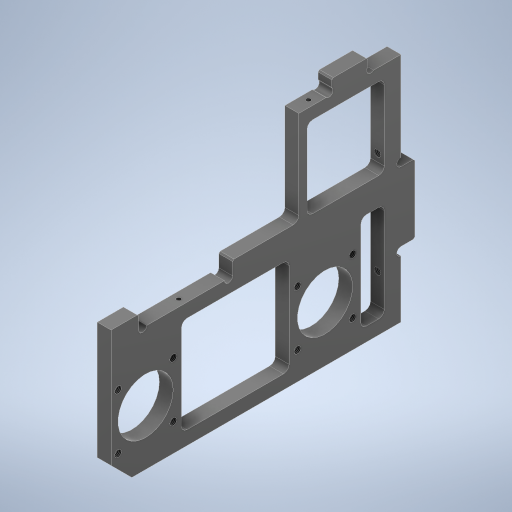
# Autodesk Inventor part: TorsoElectronicBoxSideFrame_
Saved by Autodesk Inventor 2024.2 (Build 282272000, 272)
## iProperties
Created: 2024-01-27
Part Number: TorsoElectronicBoxSideFrame_
Material: Acetal Resin, Black
Document SubType Name: Modeling
Designer: Masato Kubotera
Density: 1.425 g/cm^3
Appearance: Smooth - Black
Vendor: meviy
Mass: 35.6597 g
Surface Area: 137.332 cm^2
Volume: 25.0244 cm^3
Author: Masato Kubotera
Autodesk Inventor part; units mm, degrees
ref_plane "YZ Plane" through (0, 0, 0) normal (1, 0, 0) x (0, 1, 0)
ref_plane "XZ Plane" through (0, 0, 0) normal (0, 1, 0) x (-1, 0, 0)
ref_plane "XY Plane" through (0, 0, 0) normal (0, 0, 1) x (1, 0, 0)
derived "TorsoSideFrame.ipt"
sketch "Sketch1" plane through (0, 0, 0) normal (0, 1, 0) x (-1, 0, 0)
  circle A0 centre (0, 0) radius 18.75
  line L0 (0, 0) -> (0, -161.5)
  circle A1 centre (0, 0) radius 29 construction
  line L1 (0, 0) -> (0, 36)
  line L2 (0, 36) -> (-48.2759, 36)
  line L3 (-65, -12.5) -> (-65, -106.5)
  line L4 (-50, -161.5) -> (-35, -161.5)
  line L5 (-35, -161.5) -> (-35, -166.5)
  line L6 (-35, -166.5) -> (-10, -166.5)
  line L7 (-10, -166.5) -> (-10, -161.5)
  line L8 (-10, -161.5) -> (0, -161.5)
  line L9 (-60, -40.225) -> (-65, -40.225)
  line L10 (-44, -161.5) -> (-44, -155.5) construction
  line L11 (-22.5, -166.5) -> (-22.5, -161.5) construction
  arc A2 (-7, -161.5) -> (-10, -161.5) centre (-8.5, -161.5) ccw
  arc A3 (-35, -161.5) -> (-38, -161.5) centre (-36.5, -161.5) ccw
  line L12 (-65, -12.5) -> (-60, -12.5) construction
  line L13 (-60, -12.5) -> (-60, -101.5) construction
  line L14 (-62.5, -12.5) -> (-62.5, -101.5) construction
  line L15 (-70, -66) -> (0, -66) construction
  line L16 (-65, -40.25) -> (-60, -40.25) construction
  arc A4 (-60, -43.225) -> (-60, -40.225) centre (-60, -41.725) ccw
  line L17 (-60, -106.5) -> (0, -106.5) construction
  line L18 (-60, -101.5) -> (0, -101.5) construction
  line L19 (-60, -104) -> (-18.75, -104) construction
  line L20 (-9.95, -106.55) -> (-27.55, -106.55)
  line L21 (-27.55, -106.55) -> (-27.55, -101.45)
  line L22 (-27.55, -101.45) -> (-9.95, -101.45)
  line L23 (-9.95, -101.45) -> (-9.95, -106.55)
  line L24 (-9.95, -106.55) -> (-27.55, -101.45) construction
  line L25 (-27.55, -106.55) -> (-9.95, -101.45) construction
  line L26 (-27.5, -101.5) -> (-27.5, -106.5) construction
  arc A5 (-24.55, -101.45) -> (-27.55, -101.45) centre (-26.05, -101.45) ccw
  arc A6 (-27.55, -106.55) -> (-24.55, -106.55) centre (-26.05, -106.55) ccw
  line L27 (-22.5, -71.5) -> (-42.5, -71.5) construction
  line L28 (-42.5, -71.5) -> (-42.5, -91.5) construction
  line L29 (-42.5, -91.5) -> (-22.5, -91.5) construction
  line L30 (-22.5, -91.5) -> (-22.5, -71.5) construction
  line L31 (-22.5, -71.5) -> (-42.5, -91.5) construction
  line L32 (-42.5, -71.5) -> (-22.5, -91.5) construction
  line L33 (-45, -69) -> (-20, -69)
  line L34 (-20, -69) -> (-20, -94)
  line L35 (-20, -94) -> (-45, -94)
  line L36 (-45, -94) -> (-45, -69)
  line L37 (-45, -69) -> (-20, -94) construction
  line L38 (-20, -69) -> (-45, -94) construction
  line L39 (-50, 31) -> (0, 31) construction
  line L40 (-38.05, 31.05) -> (-13.95, 31.05)
  line L41 (-13.95, 31.05) -> (-13.95, 25.95)
  line L42 (-13.95, 25.95) -> (-38.05, 25.95)
  line L43 (-38.05, 25.95) -> (-38.05, 31.05)
  line L44 (-38.05, 31.05) -> (-13.95, 25.95) construction
  line L45 (-13.95, 31.05) -> (-38.05, 25.95) construction
  line L46 (-38.05, 28.5) -> (-13.95, 28.5) construction
  line L47 (-38, 31) -> (-38, 26) construction
  line L48 (-26, 31.05) -> (-26, 25.95) construction
  line L49 (-14, 31) -> (-14, 26) construction
  arc A7 (-35.05, 31.05) -> (-38.05, 31.05) centre (-36.55, 31.05) ccw
  arc A8 (-38.05, 25.95) -> (-35.05, 25.95) centre (-36.55, 25.95) ccw
  arc A9 (-13.95, 31.05) -> (-16.95, 31.05) centre (-15.45, 31.05) ccw
  arc A10 (-16.95, 25.95) -> (-13.95, 25.95) centre (-15.45, 25.95) ccw
  line L50 (-46.0671, -156.5) -> (-3.5, -156.5)
  arc A11 (-47.9578, -155.152) -> (-46.0671, -156.5) centre (-46.0671, -154.5) ccw
  arc A12 (-3.5, -156.5) -> (-1.5, -154.5) centre (-3.5, -154.5) ccw
  line L51 (-56, -100.25) -> (-31.1254, -100.25)
  circle A13 centre (-41.25, -65.25) radius 2 construction
  line L52 (-1.5, -63.25) -> (-56, -63.25)
  line L53 (0, 0) -> (-29, 0) construction
  line L54 (-60, -107.75) -> (-31.1254, -107.75)
  arc A14 (-29.4336, -108.6833) -> (-23.3669, -109.5167) centre (-26.05, -106.55) ccw
  line L55 (-1.5, -154.5) -> (-1.5, -109.75)
  arc A15 (-1.5, -109.75) -> (-3.5, -107.75) centre (-3.5, -109.75) ccw
  arc A16 (-29.4336, -108.6833) -> (-31.1254, -107.75) centre (-31.1254, -109.75) ccw
  circle A17 centre (-33.5, -104) radius 1.75 construction
  arc A18 (-22.0254, -109) -> (-23.3669, -109.5167) centre (-22.0254, -111) ccw
  line L56 (-18.75, -101.45) -> (-18.75, -106.55) construction
  arc A19 (-31.1254, -100.25) -> (-29.4336, -99.3167) centre (-31.1254, -98.25) ccw
  arc A20 (-23.3669, -98.4833) -> (-29.4336, -99.3167) centre (-26.05, -101.45) ccw
  arc A21 (-23.3669, -98.4833) -> (-22.0254, -99) centre (-22.0254, -97) ccw
  line L57 (-10, -101.5) -> (-10, -106.5) construction
  arc A22 (-12.95, -106.55) -> (-9.95, -106.55) centre (-11.45, -106.55) ccw
  arc A23 (-6.3746, -107.75) -> (-8.0664, -108.6833) centre (-6.3746, -109.75) ccw
  arc A24 (-14.1331, -109.5167) -> (-15.4746, -109) centre (-15.4746, -111) ccw
  arc A25 (-14.1331, -109.5167) -> (-8.0664, -108.6833) centre (-11.45, -106.55) ccw
  arc A26 (-9.95, -101.45) -> (-12.95, -101.45) centre (-11.45, -101.45) ccw
  arc A27 (-15.4746, -99) -> (-14.1331, -98.4833) centre (-15.4746, -97) ccw
  arc A28 (-8.0664, -99.3167) -> (-14.1331, -98.4833) centre (-11.45, -101.45) ccw
  arc A29 (-8.0664, -99.3167) -> (-6.3746, -100.25) centre (-6.3746, -98.25) ccw
  line L58 (-22.0254, -99) -> (-15.4746, -99)
  line L59 (-22.0254, -109) -> (-15.4746, -109)
  line L60 (-6.3746, -107.75) -> (-3.5, -107.75)
  line L61 (-6.3746, -100.25) -> (-3.5, -100.25)
  arc A30 (-3.5, -100.25) -> (-1.5, -98.25) centre (-3.5, -98.25) ccw
  line L62 (-41.25, -65.25) -> (-36.25, -65.25) construction
  line L63 (-60, -43.225) -> (-60, -87.275)
  line L64 (-60, -65.25) -> (-65, -65.25) construction
  line L65 (-65, -90.25) -> (-60, -90.25) construction
  arc A31 (-60, -90.275) -> (-60, -87.275) centre (-60, -88.775) ccw
  line L66 (-60, -90.275) -> (-65, -90.275)
  line L67 (-60, -101.5) -> (-65, -101.5) construction
  line L68 (-1.5, -22.4499) -> (-1.5, -63.25)
  line L69 (-56, -67.25) -> (-1.5, -67.25)
  line L70 (-1.5, -67.25) -> (-1.5, -98.25)
  line L71 (-56, -63.25) -> (-56, -45.4999)
  circle A32 centre (-32.5, -81.5) radius 10
  line L72 (-56, -67.25) -> (-56, -100.25)
  circle A33 centre (-32.5, -81.5) radius 11
  arc A34 (-14.0872, 17.5443) -> (-22.2374, 3.4277) centre (0, 0) ccw
  arc A35 (-22.2374, -3.4277) -> (-14.0872, -17.5443) centre (0, 0) ccw
  arc A36 (-8.1502, -20.972) -> (-1.5, -22.4499) centre (0, 0) ccw
  arc A37 (-22.2374, 3.4277) -> (-22.2374, -3.4277) centre (-24.75, 0) ccw
  line L73 (-48.2759, 36) -> (-65, -12.5)
  arc A38 (-42.9869, 36) -> (-50, 31) centre (-42.9869, 28.5817) ccw
  line L74 (-75.1102, 42.6949) -> (-93.0397, -9.3006) construction
  ellipse E0 centre (-84.0749, 16.6972) end of major axis (-76.7401, 37.9681) minor radius 15 construction
  ellipse E1 centre (-84.0749, 16.6972) end of major axis (-93.0397, -9.3006) minor radius 20 construction
  line L75 (-75.1102, 42.6949) -> (-76.7401, 37.9681) construction
  line L76 (-105, 43.5) -> (-105, 11.4504) construction
  line L77 (-84.0749, 16.6972) -> (-58.029, 7.7158) construction
  line L78 (-63.4041, 25.9649) -> (-37.3775, 16.9903) construction
  line L79 (-37.3775, 16.9903) -> (-47.4832, -12.3163) construction
  line L80 (-47.4832, -12.3163) -> (-73.5098, -3.3416) construction
  line L81 (-79.9787, 43.5) -> (-105, 43.5) construction
  line L82 (-45.1768, 19.6797) -> (-55.2826, -9.6269) construction
  circle A39 centre (-47.8663, 11.8804) radius 6.25 construction
  circle A40 centre (-52.5931, -1.8275) radius 6.25 construction
  line L83 (-1, 13.5) -> (-28, 13.5) construction
  line L84 (-28, 13.5) -> (-28, -13.5) construction
  line L85 (-28, -13.5) -> (-1, -13.5) construction
  line L86 (-1, -13.5) -> (-1, 13.5) construction
  line L87 (-1, 13.5) -> (-28, -13.5) construction
  line L88 (-28, 13.5) -> (-1, -13.5) construction
  line L89 (0, -65.25) -> (-65, -65.25) construction
  line L90 (-50, -161.5) -> (-65, -118)
  line L91 (-16.326, 23) -> (-48.5275, 23)
  arc A41 (-16.326, 23) -> (-14.0872, 17.5443) centre (-12.375, 21.4341) ccw
  line L92 (-65, -106.5) -> (-65, -118)
  arc A42 (-56, -45.4999) -> (-60, -36.225) centre (-60, -41.725) ccw
  arc A43 (-46.8371, 5.7157) -> (-50.3902, 17.5981) centre (-47.8663, 11.8804) ccw
  arc A44 (-46.8371, 5.7157) -> (-47.983, 2.3925) centre (-46.5078, 3.743) ccw
  arc A45 (-58.1048, -4.7743) -> (-47.983, 2.3925) centre (-52.5931, -1.8275) ccw
  line L93 (-48.5275, 23) -> (-50.3902, 17.5981)
  line L94 (-38, 26) -> (-14, 26) construction
  line L95 (-58.1048, -4.7743) -> (-60, -10.2703)
  line L96 (-60, -36.225) -> (-60, -10.2703)
  line L97 (-39.0921, -23.3529) -> (-39.0921, -46.6256) construction
  line L98 (-54.0921, -23.3529) -> (-54.0921, -46.6256) construction
  line L99 (-39.0921, -23.3529) -> (-54.0921, -23.3529) construction
  line L100 (-39.0921, -46.6256) -> (-54.0921, -46.6256) construction
  line L101 (-16.326, -23) -> (-48.5275, -23)
  arc A46 (-14.0872, -17.5443) -> (-16.326, -23) centre (-12.375, -21.4341) ccw
  line L102 (-47.9578, -155.152) -> (-50.3902, -148.0981)
  arc A47 (-50.3902, -148.0981) -> (-46.8371, -136.2157) centre (-47.8663, -142.3804) ccw
  arc A48 (-47.983, -132.8925) -> (-46.8371, -136.2157) centre (-46.5078, -134.243) ccw
  arc A49 (-47.983, -132.8925) -> (-58.1048, -125.7257) centre (-52.5931, -128.6725) ccw
  line L103 (-58.1048, -125.7257) -> (-60, -120.2297)
  line L104 (-60, -120.2297) -> (-60, -107.75)
  point P0 (-16.05, -9.6933)
  point P1 (-12.375, -21.4341)
  point P2 (12.375, -21.4341)
  point P3 (24.75, 0)
  point P4 (12.375, 21.4341)
  point P5 (-70, -66)
  point P6 (0, -66)
  point P7 (-47.5, -132.5)
  point P8 (-26, 28.5)
  point P9 (0, -130.75)
  point P10 (0, -158.0887)
  point P11 (-44, 28.5)
  point P12 (-61.4811, -94)
  point P13 (-1.5, -156.5)
  point P14 (-5, -161.5)
  point P15 (-29.8658, -107.75)
  point P16 (-30.0089, -107.1221)
  point P17 (-7.6342, -107.75)
  point P18 (-38, 28.5)
  point P19 (-14.5, 0)
  point P20 (-1, 0)
  point P21 (0, 22.5)
  point P22 (-62.5, -30.25)
  point P23 (-62.5, -100.25)
sketch "Sketch2" plane through (0, 0, 0) normal (0, 1, 0) x (-1, 0, 0)
  arc A0 (60, -77.75) -> (60, -80.75) centre (60, -79.25) ccw
  line L0 (60, -83.75) -> (54, -83.75) construction
  line L1 (65, -77.75) -> (60, -77.75)
  line L2 (60, -77.75) -> (60, -101.5)
  line L3 (60, -46.75) -> (54, -46.75) construction
  line L4 (60, -12.5) -> (60, -52.75)
  line L5 (65, -65.25) -> (60, -65.25) construction
  line L6 (60, -52.75) -> (65, -52.75)
  line L7 (65, -52.75) -> (65, -77.75)
  arc A1 (60, -49.75) -> (60, -52.75) centre (60, -51.25) ccw
  line L8 (60, -101.5) -> (-45, -101.5)
  line L9 (-45, -101.5) -> (-45, -51.5)
  line L10 (23, -51.5) -> (23, -12.5)
  line L11 (23, -12.5) -> (60, -12.5)
  line L12 (23, -17.5) -> (35, -17.5)
  line L13 (35, -17.5) -> (35, -12.5)
  line L14 (48, -12.5) -> (48, -17.5)
  line L15 (48, -17.5) -> (60, -17.5)
  line L16 (41.5, -12.5) -> (41.5, -17.5) construction
  arc A2 (32.8787, -17.5) -> (35, -15.3787) centre (33.9393, -16.4393) ccw
  line L17 (29, -17.5) -> (29, -23.5) construction
  arc A3 (48, -15.3787) -> (50.1213, -17.5) centre (49.0607, -16.4393) ccw
  line L18 (-35, -51.5) -> (-1, -51.5) construction
  line L19 (-1, -51.5) -> (-1, -56.5) construction
  line L20 (-1, -56.5) -> (-35, -56.5) construction
  line L21 (-35, -56.5) -> (-35, -51.5) construction
  line L22 (-35, -51.5) -> (-1, -56.5) construction
  line L23 (-1, -51.5) -> (-35, -56.5) construction
  line L24 (-35, -54) -> (-1, -54) construction
  line L25 (-18, -51.5) -> (-18, -56.5) construction
  line L26 (-0.95, -56.5) -> (-35.05, -56.5)
  line L27 (-35.05, -56.5) -> (-35.05, -51.5)
  line L28 (-0.95, -51.5) -> (-0.95, -56.5)
  arc A4 (-35.05, -56.5) -> (-32.05, -56.5) centre (-33.55, -56.5) ccw
  arc A5 (-3.95, -56.5) -> (-0.95, -56.5) centre (-2.45, -56.5) ccw
  line L29 (-60, -12.5) -> (-60, -101.5) construction
  line L30 (0, 0) -> (0, -161.5) construction
  line L31 (60, -12.5) -> (60, -101.5) construction
  line L32 (-70, -66) -> (0, -66) construction
  line L33 (-60, -101.5) -> (0, -101.5) construction
  line L34 (-65, -12.5) -> (-60, -12.5) construction
  line L35 (26, -22) -> (26, -51.5)
  line L36 (26, -51.5) -> (54, -51.5)
  line L37 (54, -51.5) -> (54, -22)
  line L38 (54, -22) -> (26, -22)
  line L39 (-45, -51.5) -> (-35.05, -51.5)
  line L40 (23, -51.5) -> (-0.95, -51.5)
  line L41 (45.5, -61.5) -> (54, -61.5)
  line L42 (54, -61.5) -> (54, -96.5)
  line L43 (54, -96.5) -> (45.5, -96.5)
  line L44 (45.5, -96.5) -> (45.5, -61.5)
  circle A6 centre (-32.5, -81.5) radius 10 projected
  circle A7 centre (32.5, -81.5) radius 10
  line L45 (-19.5, -61.5) -> (19.5, -61.5)
  line L46 (19.5, -61.5) -> (19.5, -96.5)
  line L47 (19.5, -96.5) -> (-19.5, -96.5)
  line L48 (-19.5, -96.5) -> (-19.5, -61.5)
  circle A8 centre (-22.5, -71.5) radius 3 construction
  circle A9 centre (42.5, -71.5) radius 3 construction
  point P0 (-18, -54)
  point P1 (-41, -54)
  point P2 (5, -54)
  point P3 (-42.5, -71.5)
  point P4 (-42.5, -91.5)
  point P5 (-22.5, -91.5)
  point P6 (42.5, -91.5)
  point P7 (22.5, -91.5)
  point P8 (22.5, -71.5)
  point P9 (-0.95, -56.5)
  point P10 (-3.95, -56.5)
  point P11 (-30.05, -61.55)
  point P12 (-30.05, -61.55)
  point P13 (50.1213, -17.5)
  point P14 (48, -15.3787)
  point P15 (-0.95, -56.5)
  dimension "d1" = 25
  dimension "d2" = 6
  dimension "d3" = 1.5
  dimension "d5" = 6
  dimension "d7" = 5
  dimension "d8" = 6
  dimension "d9" = 6
  dimension "d11" = 5
  dimension "d13" = 0.05
  dimension "d15" = 6
  dimension "d19" = 25
  dimension "d20" = 15
  dimension "d21" = 45
  dimension "d22" = 5
  dimension "d23" = 34
  dimension "d24" = 37
  dimension "d64" = 3
  dimension "d65" = 12
  dimension "d68" = 4.5
  dimension "d69" = 89
  dimension "d71" = 52.75
  dimension "d80" = 5
  dimension "d81" = 5
  dimension "d82" = 6
  constraints: 88 end point, 18 symmetric about line, 16 point on line, 14 horizontal, 13 point on circle, 11 collinear, 9 centre point, 9 midpoint, 8 vertical, 6 parallel, 6 perpendicular, 3 equal radius, 3 tangent, 2 coincident, 8 other
  measures "d1" distance of L7.start L7.end
  measures "d2" distance of L3.start L3.end
  measures "d3" radius of A1
  measures "d5" distance between parallel lines of L3 L6
  measures "d7" distance between parallel lines of L12 L11
  measures "d8" distance of L17.start L17.end
  measures "d9" distance between parallel lines of L13 L17
  measures "d11" distance of L18.end L20.start
  measures "d13" distance between parallel lines of L27 L21
  measures "d15" distance from line of point (-41, -54) L21
  measures "d19" distance between parallel lines of L21 L29
  measures "d20" distance between parallel lines of L29 L9
  measures "d21" distance between parallel lines of L8 L20
  measures "d22" distance of L7.end L2.start
  measures "d23" distance between parallel lines of L21 L19
  measures "d24" distance of L11.start L4.start
  measures "d64" distance between parallel lines of L10 L35
  measures "d65" distance between parallel lines of L10 L13
  measures "d68" distance between parallel lines of L38 L12
  measures "d69" distance between parallel lines of L8 L11
  measures "d71" vertical distance of L5.start L4.start
  measures "d80" distance between parallel lines of L45 L20
  measures "d81" distance between parallel lines of L33 L47
  measures "d82" diameter of A8
extrude "Extrusion1" add sketch "Sketch2" against normal blind 5 contours A0 L2 L8 L9 L39 L27 A4 L26 A5 L28 L40 L10 L12 A2 L13 L11 L14 A3 L15 L4 A1 L6 L7 L1
hole "M3" at (42.5, 0, -71.5) at (42.5, 0, -91.5) at (22.5, 0, -91.5) at (22.5, 0, -71.5) at (-22.5, 0, -71.5) at (-22.5, 0, -91.5) at (-42.5, 0, -91.5) at (-42.5, 0, -71.5) direction (0, -1, 0) diameter 2.459 end through all thread size "M3x0.5" class "6H" standard "ANSI Metric M Profile"
sketch "Sketch3" plane through (-60, 0, -49.75) normal (-1, 0, 0) x (0, 0, -1)
  line L0 (3, 5) -> (0, 5) projected
  line L1 (-3, 5) -> (-3, 0)
  line L2 (28, 5) -> (51.75, 5) projected
  line L3 (34, 5) -> (34, 0)
  point P0 (-49.75, 0)
  point P1 (-32.25, 5)
  point P2 (31, 5)
  point P3 (-3, 0)
  point P4 (-3, 0)
  point P5 (-3, 0)
  point P6 (34, 0)
  point P7 (34, 0)
  point P8 (34, 0)
  point P9 (-3, 2.5)
  point P10 (34, 2.5)
  point P11 (-49.25, 5)
  constraints: 4 end point, 2 coincident, 2 midpoint, 2 point on line, 2 vertical
hole "Side-M3" at (-60, -2.5, -46.75) at (-60, -2.5, -83.75) direction (1, 0, 0) diameter 2.459 depth 6 thread size "M3x0.5" class "6H" standard "ANSI Metric M Profile"
sketch "Sketch4" plane through (-32.8787, 0, -17.5) normal (0, 0, 1) x (-1, 0, 0)
  line L0 (-9.8787, 5) -> (0, 5) projected
  line L1 (-3.8787, 5) -> (-3.8787, 0)
  point P0 (-32.8787, 0)
  point P1 (-3.8787, 0)
  point P2 (-3.8787, 0)
  point P3 (-3.8787, 0)
  point P4 (-3.8787, 2.5)
  constraints: 2 end point, 1 coincident, 1 midpoint, 1 point on line, 1 vertical
hole "Top-M3" at (-29, -2.5, -17.5) direction (0, 0, -1) diameter 1.567 depth 6 thread size "M2x0.4" class "6H" standard "ANSI Metric M Profile"
sketch "Sketch5" plane through (3.95, 0, -56.5) normal (0, 0, 1) x (1, 0, 0)
  line L0 (14.05, -5) -> (14.05, 0)
  line L1 (0, 0) -> (28.1, 0) projected
  line L2 (28.1, -5) -> (0, -5) projected
  point P0 (-3.95, 0)
  point P1 (14.05, -2.5)
  constraints: 3 midpoint, 2 end point
hole "Top-M2" at (18, -2.5, -56.5) direction (0, 0, -1) diameter 1.567 depth 6 thread size "M2x0.4" class "6H" standard "ANSI Metric M Profile"
fillet "R2" radius 2 13 edges at (-23, -2.5, -51.5) (-26, -2.5, -51.5) (-26, -2.5, -22) (-54, -2.5, -22) (-54, -2.5, -51.5) (19.5, -2.5, -61.5) (-19.5, -2.5, -61.5) (-19.5, -2.5, -96.5) (19.5, -2.5, -96.5) (-45.5, -2.5, -61.5) (-54, -2.5, -61.5) (-45.5, -2.5, -96.5) (-54, -2.5, -96.5)
chamfer "C0.5" distance 0.5 angle 45 6 edges at (-48, -2.5, -12.5) (-35, -2.5, -12.5) (-65, -2.5, -52.75) (-65, -2.5, -77.75) (35.05, -2.5, -51.5) (0.95, -2.5, -51.5)
chamfer "C7.5" distance 7.5 angle 45 1 edges at (45, -2.5, -101.5)
equation "\"d49\" = d2"
body "Solid1"
